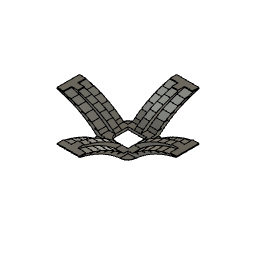
bear_overhang_small_50-75 (Autodesk Fusion 360 design; units mm, degrees)
Autodesk Fusion 360 part; units mm, degrees
sketch "arm" plane through (0, 0, 0) normal (0, 1, 0) x (1, 0, 0) in component "bear_overhang_small_50-75"
  line L0 (15, 0) -> (10, 0)
  line L1 (24.3844, -7.2) -> (29.5805, -10.2)
  line L2 (15, 0) -> (19.5287, -3.8)
  line L3 (19.5287, -3.8) -> (24.3844, -7.2)
  line L4 (0, -2) -> (0, 0)
  line L5 (0, 0) -> (0, -27.1786) construction
  line L6 (24.5805, -10.2) -> (19.3844, -7.2)
  line L7 (29.5805, -10.2) -> (24.5805, -10.2) construction
  line L8 (24.3844, -7.2) -> (19.3844, -7.2) construction
  line L9 (19.5287, -3.8) -> (14.5287, -3.8) construction
  line L10 (19.3844, -7.2) -> (14.5287, -3.8)
  line L11 (14.5287, -3.8) -> (10, 0)
  line L12 (29.5805, -10.2) -> (35.1562, -12.8)
  line L13 (35.1562, -12.8) -> (40.6512, -14.8)
  line L14 (24.5805, -10.2) -> (30.1562, -12.8)
  line L15 (30.1562, -12.8) -> (35.6512, -14.8)
  line L16 (35.1562, -12.8) -> (30.1562, -12.8) construction
  line L17 (10, 0) -> (0, 0)
  line L18 (0, -2) -> (12.3835, -2)
  line L19 (7.3835, -2) -> (9.5287, -3.8)
  line L20 (9.5287, -3.8) -> (14.3844, -7.2)
  line L21 (14.3844, -7.2) -> (19.5805, -10.2)
  line L22 (19.5805, -10.2) -> (25.1562, -12.8)
  line L23 (25.1562, -12.8) -> (30.6512, -14.8)
  line L24 (40.6512, -14.8) -> (46.6225, -16.4)
  line L25 (46.6225, -16.4) -> (41.6225, -16.4)
  line L26 (41.6225, -16.4) -> (36.6225, -16.4)
  line L27 (36.6225, -16.4) -> (30.6512, -14.8)
  line L28 (35.6512, -14.8) -> (40.6512, -14.8) construction
  line L29 (35.6512, -14.8) -> (41.6225, -16.4)
  line L30 (36.6225, -16.4) -> (36.6225, -17)
  line L31 (36.6225, -17) -> (46.6225, -17)
  line L32 (46.6225, -17) -> (46.6225, -16.4)
  line L33 (41.6225, -16.4) -> (41.6225, -17)
  dimension "d9" = 3.8
  dimension "d10" = 3.4
  dimension "d13" = 3
  dimension "d24" = 50
  dimension "d25" = 55
  dimension "d26" = 60
  dimension "d45" = 7.6
  dimension "d46" = 7.6019
  dimension "d50" = 65
  dimension "d51" = 70
  dimension "d52" = 2.6
  dimension "d53" = 2
  dimension "d54" = 6.6254
  dimension "d55" = 7.0171
  dimension "d78" = 5
  dimension "d79" = 10
  dimension "d84" = 2
  dimension "d85" = 5.9118
  dimension "d98" = 5
  dimension "d99" = 75
  dimension "d100" = 10.1153
  dimension "d101" = 1.6
  dimension "d105" = 0.6
  constraint horizontal L7
  constraint horizontal L8
  constraint horizontal L9
  constraint horizontal L0
  constraint coincident L4.end L5.start
  constraint horizontal L16
  constraint perpendicular L5 L17
  constraint parallel L0 L17
  constraint equal L0 L9
  constraint perpendicular L4 L17
  constraint coincident L11 L18.end
  constraint perpendicular L5 L18
  constraint coincident L18 L19.start
  constraint parallel L11 L19
  constraint parallel L10 L20
  constraint parallel L6 L21
  constraint parallel L14 L22
  constraint coincident L9 L19.end
  constraint coincident L7 L21.end
  constraint coincident L8 L20.end
  constraint parallel L15 L23
  constraint coincident L16 L22.end
  constraint horizontal L28
  constraint coincident L23.end L28
  constraint horizontal L25
  constraint parallel L27 L29
  constraint parallel L25 L26
  constraint equal L8 L9
  constraint equal L7 L8
  constraint equal L7 L16
  constraint equal L16 L28
  constraint equal L25 L28
  constraint perpendicular L26 L30
  constraint perpendicular L30 L31
  constraint perpendicular L25 L32
  constraint perpendicular L31 L33
  constraint coincident L31 L33.end
  measures "d9" vertical distance of L2.end L0.start
  measures "d10" vertical distance of L2.end L1.start
  measures "d13" vertical distance of L1.end L1.start
  measures "d24" angle of L2 L5
  measures "d25" angle of L3 L5
  measures "d26" angle of L1 L5
  measures "d50" angle of L5 L12
  measures "d51" angle of L5 L13
  measures "d52" vertical distance of L1.end L12.end
  measures "d53" vertical distance of L13.end L12.end
  measures "d78" distance of L0.start L0.end
  measures "d79" distance of L4.end L0.end
  measures "d84" distance of L4.end L4.start
  measures "d85" distance of L2.end L0.start
  measures "d98" distance of L18.end L19.start
  measures "d99" angle of L5 L24
  measures "d101" vertical distance of L13.end L24.end
  measures "d105" distance of L24.end L31.end
extrude "Extrude1" add sketch "arm" along normal mid plane 18 contours L0 L1 L2 L3 L6 L10 L11 L12 L13 L14 L15 L24 L25 L29 | L4 L11 L17 L18 | L25 L31 L32 L33 makes body 1 in component "bear_overhang_small_50-75"
extrude "Extrude2" add sketch "arm" along normal mid plane 5 contours L6 L10 L11 L14 L15 L18 L19 L20 L21 L22 L23 L26 L27 L29 | L26 L30 L31 L33 bodies 1 in component "bear_overhang_small_50-75"
sketch "angle_indication" plane through (0, -9, 0) normal (0, -1, 0) x (1, 0, 0) in component "bear_overhang_small_50-75"
  line L0 (19.5287, 3.8) -> (14.5287, 3.8)
  line L1 (24.3844, 7.2) -> (19.3844, 7.2)
  line L2 (29.5805, 10.2) -> (24.5805, 10.2)
  line L3 (35.1562, 12.8) -> (30.1562, 12.8)
  line L4 (17.0287, 3.8) -> (17.3143, 4)
  line L5 (17.3143, 4) -> (14.8143, 4)
  line L6 (21.8844, 7.2) -> (22.2308, 7.4)
  line L7 (22.2308, 7.4) -> (19.7308, 7.4)
  line L8 (27.0805, 10.2) -> (27.5094, 10.4)
  line L9 (27.5094, 10.4) -> (25.0094, 10.4)
  line L10 (32.6562, 12.8) -> (33.2057, 13)
  line L11 (33.2057, 13) -> (30.7057, 13)
  line L12 (19.3844, 7.2) -> (14.5287, 3.8)
  line L13 (24.5805, 10.2) -> (19.3844, 7.2)
  line L14 (30.1562, 12.8) -> (24.5805, 10.2)
  line L15 (35.6512, 14.8) -> (30.1562, 12.8)
  line L16 (41.6225, 16.4) -> (35.6512, 14.8)
  line L17 (40.6512, 14.8) -> (35.6512, 14.8)
  line L18 (36.3976, 15) -> (38.8976, 15)
  line L19 (38.8976, 15) -> (38.1512, 14.8)
  line L20 (46.6225, 17) -> (41.6225, 17)
  line L21 (41.6225, 17) -> (41.6225, 16.4)
  line L22 (46.6225, 16.4) -> (46.6225, 17)
  line L23 (41.6225, 16.4) -> (46.6225, 16.4)
  point P0 (19.5287, 3.8)
  point P1 (24.3844, 7.2)
  point P2 (29.5805, 10.2)
  point P3 (35.1562, 12.8)
  point P4 (40.6512, 14.8)
  dimension "d68" = 0.2
  dimension "d69" = 0.2
  dimension "d70" = 0.2
  dimension "d71" = 0.2
  dimension "d102" = 0.2
  constraint midpoint L0 L4.start
  constraint midpoint L1 L6.start
  constraint midpoint L2 L8.start
  constraint midpoint L3 L10.start
  constraint parallel L0 L5
  constraint parallel L1 L7
  constraint parallel L2 L9
  constraint parallel L3 L11
  constraint coincident L11.end L15
  constraint coincident L3.end L14.start
  constraint coincident L2.end L13.start
  constraint coincident L1.end L12.start
  constraint coincident L0.end L12.end
  constraint parallel L4 L12
  constraint parallel L6 L13
  constraint parallel L8 L14
  constraint parallel L10 L15
  constraint coincident L9.end L14
  constraint coincident L7.end L13
  constraint coincident L5.end L12
  constraint coincident P0 L0.start
  constraint coincident P1 L1.start
  constraint coincident P2 L2.start
  constraint coincident P3 L3.start
  constraint coincident P4 L17.start
  constraint coincident L15.start L16.end
  constraint coincident L16 L18.start
  constraint parallel L17 L18
  constraint midpoint L17 L19.end
  constraint parallel L16 L19
  constraint coincident L16.start L21.end
  constraint coincident L22.start L23.end
  measures "d68" distance of L0 L5
  measures "d69" distance of L1 L7
  measures "d70" distance of L2 L9
  measures "d71" distance of L3 L11
  measures "d102" distance of L17 L18
extrude "Extrude2'" cut sketch "angle_indication" against normal blind 0.3 bodies 1 in component "bear_overhang_small_50-75"
mirror "Mirror1" about plane through (0, 0, 0) normal (0, 1, 0) of "Extrude2'" in component "bear_overhang_small_50-75"
pattern_circular "C-Pattern1" count 4 over 360 about axis through (0, 0, 1.75) along (0, 0, 1) of bodies 1 makes body 2 at (0.8333, 2.4612, 2) makes body 3 at (-44.9558, -0.8333, 17) makes body 4 at (3, -5, 0) in component "bear_overhang_small_50-75"
combine "Combine1" operation add target body 1 tool bodies 4 3 2 in component "bear_overhang_small_50-75"
sketch "orientation_mark" plane through (0, 0, 0) normal (0, 0, -1) x (1, 0, 0) in component "bear_overhang_small_50-75"
  line L0 (-9, 9) -> (-15, 9)
  line L1 (9, -9) -> (15, -9)
  line L2 (-9, -9) -> (-9, -15)
  line L3 (9, -15) -> (9, -9)
  line L4 (15, 9) -> (9, 9)
  line L5 (9, 9) -> (9, 15)
  line L6 (-9, 15) -> (-9, 9)
  arc A0 (9, -15) -> (15, -9) centre (9, -9) ccw
  arc A1 (15, 9) -> (9, 15) centre (9, 9) ccw
  arc A2 (-9, 15) -> (-15, 9) centre (-9, 9) ccw
  arc A3 (-15, -9) -> (-9, -15) centre (-9, -9) ccw
  line L7 (-15, 9) -> (-15, -9)
  line L8 (-9, -15) -> (9, -15)
  line L9 (15, -9) -> (15, 9)
  line L10 (9, 15) -> (-9, 15)
  line L11 (-15, -9) -> (-9, -9)
  line L12 (0, 15) -> (0, -15) construction
  line L13 (-15, 0) -> (15, 0) construction
  line L14 (-7.3835, -2.5) -> (-7.3835, 2.5)
  line L15 (-2.5, 7.3835) -> (2.5, 7.3835)
  line L16 (7.3835, 2.5) -> (7.3835, -2.5)
  line L17 (2.5, -7.3835) -> (-2.5, -7.3835)
  line L18 (-7.3835, -2.5) -> (-7.3835, -7.3835)
  line L19 (-7.3835, -7.3835) -> (-2.5, -7.3835)
  line L20 (2.5, -7.3835) -> (7.3835, -7.3835)
  line L21 (7.3835, -7.3835) -> (7.3835, -2.5)
  line L22 (2.5, 7.3835) -> (7.3835, 7.3835)
  line L23 (7.3835, 7.3835) -> (7.3835, 2.5)
  arc A4 (-2.5, 7.3835) -> (-7.3835, 2.5) centre (-2.5, 2.5) ccw
  constraint coincident L2.end A3.end
  constraint coincident A3.start L7.end
  constraint coincident L0.end A2.end
  constraint coincident L6.start A2.start
  constraint coincident L5.end A1.end
  constraint coincident L1.end A0.end
  constraint coincident L3.start A0.start
  constraint tangent A0 L8
  constraint tangent A3 L8
  constraint tangent A2 L7
  constraint tangent A1 L10
  constraint coincident L4.start A1.start
  constraint midpoint L10 L12.start
  constraint midpoint L8 L12.end
  constraint midpoint L7 L13.start
  constraint midpoint L9 L13.end
  constraint coincident L14.start L18.start
  constraint parallel L14 L18
  constraint coincident L17.end L19.end
  constraint coincident L17.start L20.start
  constraint parallel L17 L20
  constraint coincident L16.end L21.end
  constraint parallel L16 L21
  constraint parallel L17 L19
  constraint coincident L15.end L22.start
  constraint parallel L15 L22
  constraint coincident L16.start L23.end
  constraint parallel L16 L23
  constraint tangent L15 A4
  constraint tangent L14 A4
  constraint coincident L15.start A4.start
  constraint coincident L14.end A4.end
extrude "Extrude3" add sketch "orientation_mark" against normal blind 0.2 contours L0 L6 A2 | L2 A3 L11 | L4 L5 A1 | L1 L3 A0 bodies 1 in component "bear_overhang_small_50-75"
extrude "Extrude4" cut sketch "orientation_mark" along normal up to surface (2 mm away) from surface at -2 contours L14 L15 L16 L17 L18 L19 L20 L21 L22 L23 A4 bodies 1 in component "bear_overhang_small_50-75"
component "bear_overhang_small_50-75" placed x (1, 0, 0) y (0, 1, 0) z (0, 0, 1) at (0, 0, 0)
equation "d9 = layer_height * 19"
equation "d10 = layer_height * 17"
equation "d13 = layer_height * 15"
equation "d31 = arm_width"
equation "layer_height = 0.2 mm"
equation "arm_width = 18 mm"
equation "arm_support_width = arm_width / 3"
equation "d52 = layer_height * 13"
equation "d53 = layer_height * 10"
equation "arm_layer_length = e_width + ( num_perimeters * 2 - 1 ) * e_spacing"
equation "d68 = layer_height"
equation "d69 = layer_height"
equation "d70 = layer_height"
equation "d71 = layer_height"
equation "d75 = -layer_height"
equation "e_width = 0.45 mm"
equation "e_spacing = 0.4071 mm"
equation "num_perimeters = 2"
equation "d101 = layer_height * 8"
equation "d102 = layer_height"
equation "num_bottom_layers = 4"
equation "num_top_layers = 3"
equation "d105 = num_top_layers * layer_height"
